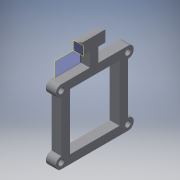
# Autodesk Inventor part: back_pack_side_clip_in
Saved by Autodesk Inventor 2016 (Build 200138000, 138)
## iProperties
Created: 2016-05-19
Part Number: back_pack_side_clip_in
Material: Generic
Document SubType Name: Modeling
Designer: ajar021
Density: 1 g/cm^3
Appearance: Default
Author: ajar021
Autodesk Inventor part; units mm, degrees
ref_plane "Work Plane1" through (11, 2.9624, 8) normal (0, 0, -1) x (-1, 0, 0)
sketch "Sketch1" plane through (11, 2.9624, 8) normal (0, 0, -1) x (-1, 0, 0)
  arc A0 (0.0647, 1) -> (3.5, -0.2722) centre (5.5324, 10.4896) ccw projected
  line L0 (0, -2.9624) -> (0, 1) projected
  line L1 (3.5, -0.2722) -> (3.5, -2.9624) projected
  line L2 (0, -2.9624) -> (3.5, -2.9624) projected
  arc A1 (0, 1.0376) -> (11, 1) centre (5.5324, 10.4896) ccw projected
  line L3 (0, -7.9624) -> (0, 1.0376) projected
  line L4 (3.5, -0.2722) -> (3.5, -2.9624)
  line L5 (0, -2.9624) -> (3.5, -2.9624)
  line L6 (0, -2.9624) -> (0, 1.0376)
  arc A2 (0, 1.0376) -> (11, 1) centre (5.5324, 10.4896) ccw
  point P0 (11, -2.9624)
  constraints: 6 end point, 2 collinear, 2 point on circle, 1 centre point, 1 perpendicular, 4 other
ref_plane "Work Plane2" through (8, 0, 0) normal (0, 0, 1) x (1, 0, 0)
ref_plane "Work Plane4" through (8, 0, 0) normal (0, 0, 1) x (1, 0, 0)
extrude "Extrusion1" add sketch "Sketch1" along normal up to surface (8 mm away)
ref_plane "Work Plane3" through (8, -5, 14.5) normal (-1, 0, 0) x (0, 0, 1)
ref_plane "Work Plane5" through (11, -5, -9) normal (1, 0, 0) x (0, 1, 0)
sketch "Sketch2" plane through (8, -5, 14.5) normal (-1, 0, 0) x (0, 0, 1)
  line L0 (-6.5, 5) -> (-14.5, 5) projected
  line L1 (-12, 5) -> (-12, 0) projected
  line L2 (-12, 5) -> (-12, 0)
  line L3 (-12, 5) -> (-9.4556, 5)
  line L4 (-12, 0) -> (-22.5, 0)
  line L5 (-22.5, 0) -> (-22.5, -26)
  line L6 (1.0444, 0) -> (1.0444, -26)
  line L7 (1.0444, -26) -> (-22.5, -26)
  line L8 (-22.5, 0) -> (-19.5, 0)
  line L9 (-19.5, 0) -> (-19.5, -3)
  line L10 (1.0444, -26) -> (1.0444, -23)
  line L11 (1.0444, -23) -> (-1.9556, -23)
  line L12 (-19.5, -3) -> (-1.9556, -3)
  line L13 (-1.9556, -3) -> (-1.9556, -23)
  line L14 (-1.9556, -23) -> (-19.5, -23)
  line L15 (-19.5, -23) -> (-19.5, -3)
  line L16 (1.0444, -26) -> (-0.9556, -26)
  line L17 (-0.9556, -26) -> (-2.9556, -26)
  line L18 (-22.5, 0) -> (-22.5, -4)
  line L19 (-22.5, -4) -> (-22.5, -2)
  line L20 (-22.5, -2) -> (-24.5, -2)
  line L21 (1.0444, 0) -> (1.0444, -4)
  line L22 (1.0444, -2) -> (3.0444, -2)
  arc A0 (-22.5, 0) -> (-22.5, -4) centre (-22.5, -2) ccw
  arc A1 (1.0444, -4) -> (1.0444, 0) centre (1.0444, -2) ccw
  line L23 (-9, 0) -> (-9, 5) projected
  line L24 (-12, 5) -> (-9, 5)
  line L25 (-9, 5) -> (-9, 0)
  line L26 (1.0444, 0) -> (-9, 0)
  line L27 (-22.5, -26) -> (-22.5, -24)
  line L28 (-22.5, -24) -> (-24.5, -24)
  line L29 (1.0444, -26) -> (1.0444, -24)
  line L30 (1.0444, -24) -> (3.0444, -24)
  line L31 (-22.5, -24) -> (-22.5, -22)
  line L32 (1.0444, -24) -> (1.0444, -22)
  arc A2 (-22.5, -22) -> (-22.5, -26) centre (-22.5, -24) ccw
  arc A3 (1.0444, -26) -> (1.0444, -22) centre (1.0444, -24) ccw
  line L33 (-19.5, -23) -> (-1.9556, -23)
  line L34 (-1.9556, -3) -> (-1.9556, -23)
  point P0 (-18.5, -26)
  dimension "d3" = 10.5
  dimension "d4" = 26
  dimension "d5" = 3
  dimension "d6" = 3
  dimension "d8" = 3
  dimension "d16" = 4
  dimension "d17" = 2
  dimension "d18" = 4
  dimension "d19" = 2
  dimension "d28" = 2
  dimension "d29" = 2
  dimension "d30" = 2
  dimension "d31" = 2
  dimension "d32" = 2
  constraints: 64 end point, 12 point on circle, 12 point on line, 8 perpendicular, 5 collinear, 4 centre point, 4 horizontal, 2 midpoint, 2 parallel, 2 vertical, 1 tangent
  measures "d3" distance of L1.end L4.end
  measures "d4" distance of L4.end L5.end
  measures "d5" distance of L4.end L8.end
  measures "d6" distance of L8.end L9.end
  measures "d8" distance of L10.end L11.end
  measures "d16" distance of L4.end L18.end
  measures "d17" distance of L19.end L20.end
  measures "d18" distance of L6.start L21.end
  measures "d19" distance of L22.start L22.end
  measures "d28" distance of L5.end L27.end
  measures "d29" distance of L29.end L30.end
  measures "d30" distance of L6.end L29.end
  measures "d31" distance of L27.end L31.end
  measures "d32" distance of L29.end L32.end
extrude "Extrusion2" add sketch "Sketch2" along normal up to surface (3.5 mm away) from surface at -3 contours L23 L26 L6 L11 L13 L12 L9 L4 L1 L0 | A1 L22 L6 | L22 A1 L6 | L9 L15 L14 L11 L6 L7 L5 L4 | L5 L20 A0 | A3 L30 L6 | L5 A0 L20 | A3 L6 L30 | L5 L28 A2 | L5 A2 L28
sketch "Sketch3" plane through (11, 0, 8) normal (1, 0, 0) x (0, 0, -1)
  arc A0 (-7.5444, -5) -> (-7.5444, -9) centre (-7.5444, -7) ccw projected
  arc A1 (16, -9) -> (16, -5) centre (16, -7) ccw projected
  circle A2 centre (16, -7) radius 1
  circle A3 centre (-7.5444, -7) radius 1
  arc A4 (-7.5444, -27) -> (-7.5444, -31) centre (-7.5444, -29) ccw projected
  arc A5 (16, -31) -> (16, -27) centre (16, -29) ccw projected
  circle A6 centre (16, -29) radius 1
  circle A7 centre (-7.5444, -29) radius 1
  point P0 (-5.5444, -31)
  dimension "d23" = 2
  dimension "d25" = 2
  dimension "d33" = 2
  dimension "d34" = 2
  constraints: 4 centre point, 4 coincident
  measures "d23" diameter of A2
  measures "d25" diameter of A3
  measures "d33" diameter of A6
  measures "d34" diameter of A7
extrude "Extrusion3" cut sketch "Sketch3" against normal up to surface (3.5 mm away)
body "Solid1"
